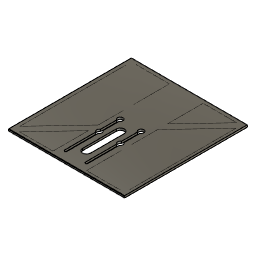
GuG_Back (Autodesk Fusion 360 design; units mm, degrees)
Autodesk Fusion 360 part; units mm, degrees
sketch "Sketch1" plane through (0, 0, 0) normal (0, 0, 1) x (1, 0, 0)
  line L0 (86.5, 91.5) -> (-86.5, 91.5)
  line L1 (-86.5, 91.5) -> (-86.5, -91.5)
  line L2 (-86.5, -91.5) -> (86.5, -91.5)
  line L3 (86.5, -91.5) -> (86.5, 91.5)
  line L4 (86.5, 91.5) -> (-86.5, -91.5) construction
  line L5 (-86.5, 91.5) -> (86.5, -91.5) construction
  line L6 (0, -91.5) -> (0, -61.5)
  line L7 (15.5, -77) -> (-15.5, -77)
  line L8 (-15.5, -77) -> (-15.5, -46)
  line L9 (-15.5, -46) -> (15.5, -46)
  line L10 (15.5, -46) -> (15.5, -77)
  line L11 (15.5, -77) -> (-15.5, -46) construction
  line L12 (-15.5, -77) -> (15.5, -46) construction
  circle A0 centre (-15.5, -77) radius 1.75
  circle A1 centre (-15.5, -46) radius 1.75
  circle A2 centre (15.5, -46) radius 1.75
  circle A3 centre (15.5, -77) radius 1.75
  line L13 (0, -61.5) -> (0, -11.5)
  line L14 (15.5, -27) -> (-15.5, -27)
  line L15 (-15.5, -27) -> (-15.5, 4)
  line L16 (-15.5, 4) -> (15.5, 4)
  line L17 (15.5, 4) -> (15.5, -27)
  line L18 (15.5, -27) -> (-15.5, 4) construction
  line L19 (-15.5, -27) -> (15.5, 4) construction
  circle A4 centre (-15.5, 4) radius 1.75
  circle A5 centre (15.5, 4) radius 1.75
  circle A6 centre (15.5, -27) radius 1.75
  circle A7 centre (-15.5, -27) radius 1.75
  circle A8 centre (-15.5, 4) radius 4
  circle A9 centre (15.5, 4) radius 4
  circle A10 centre (0, -61.5) radius 6
  circle A11 centre (0, -11.5) radius 6
  line L20 (13.75, 4) -> (17.25, 4)
  line L21 (17.25, 4) -> (17.25, -77)
  line L22 (17.25, -77) -> (13.75, -77)
  line L23 (13.75, -77) -> (13.75, 4)
  line L24 (-13.75, 4) -> (-17.25, 4)
  line L25 (-17.25, 4) -> (-17.25, -77)
  line L26 (-17.25, -77) -> (-13.75, -77)
  line L27 (-13.75, -77) -> (-13.75, 4)
  line L28 (-6, -11.5) -> (6, -11.5)
  line L29 (6, -11.5) -> (6, -61.5)
  line L30 (6, -61.5) -> (-6, -61.5)
  line L31 (-6, -61.5) -> (-6, -11.5)
  line L32 (25, -91.5) -> (-25, -91.5)
  line L33 (-25, -91.5) -> (-25, 91.5)
  line L34 (-25, 91.5) -> (25, 91.5)
  line L35 (25, 91.5) -> (25, -91.5)
  line L36 (25, -91.5) -> (-25, 91.5) construction
  line L37 (-25, -91.5) -> (25, 91.5) construction
  line L38 (-86.5, -91.5) -> (86.5, 91.5)
  line L39 (86.5, 91.5) -> (82.8666, 94.9349)
  line L40 (82.8666, 94.9349) -> (-90.1334, -88.0651)
  line L41 (-90.1334, -88.0651) -> (-86.5, -91.5)
  line L42 (-86.5, -91.5) -> (86.5, 91.5)
  line L43 (86.5, 91.5) -> (90.1334, 88.0651)
  line L44 (90.1334, 88.0651) -> (-82.8666, -94.9349)
  line L45 (-82.8666, -94.9349) -> (-86.5, -91.5)
  line L46 (86.5, -91.5) -> (-86.5, 91.5)
  line L47 (-86.5, 91.5) -> (-82.8666, 94.9349)
  line L48 (-82.8666, 94.9349) -> (90.1334, -88.0651)
  line L49 (90.1334, -88.0651) -> (86.5, -91.5)
  line L50 (86.5, -91.5) -> (-86.5, 91.5)
  line L51 (-86.5, 91.5) -> (-90.1334, 88.0651)
  line L52 (-90.1334, 88.0651) -> (82.8666, -94.9349)
  line L53 (82.8666, -94.9349) -> (86.5, -91.5)
  line L54 (81.5, -86.5) -> (-81.5, -86.5)
  line L55 (-81.5, -86.5) -> (-81.5, 86.5)
  line L56 (-81.5, 86.5) -> (81.5, 86.5)
  line L57 (81.5, 86.5) -> (81.5, -86.5)
  line L58 (81.5, -86.5) -> (-81.5, 86.5) construction
  line L59 (-81.5, -86.5) -> (81.5, 86.5) construction
  circle A12 centre (-15.5, -27) radius 4
  circle A13 centre (15.5, -27) radius 4
  point P0 (0, -91.5)
  point P1 (0, -61.5)
  point P2 (0, -11.5)
  dimension "d1" = 173
  dimension "d2" = 183
  dimension "d3" = 30
  dimension "d4" = 31
  dimension "d5" = 31
  dimension "d6" = 3.5
  dimension "d7" = 3.5
  dimension "d8" = 3.5
  dimension "d9" = 3.5
  dimension "d10" = 50
  dimension "d11" = 31
  dimension "d12" = 31
  dimension "d13" = 3.5
  dimension "d14" = 3.5
  dimension "d15" = 3.5
  dimension "d16" = 3.5
  dimension "d17" = 8
  dimension "d18" = 8
  dimension "d19" = 12
  dimension "d20" = 12
  dimension "d21" = 3.5
  dimension "d22" = 3.5
  dimension "d31" = 50
  dimension "d32" = 5
  dimension "d33" = 5
  dimension "d34" = 5
  dimension "d35" = 5
  dimension "d36" = 163
  dimension "d37" = 173
  dimension "d42" = 8
  dimension "d43" = 8
  constraint horizontal L0
  constraint perpendicular L0 L1
  constraint parallel L0 L2
  constraint parallel L1 L3
  constraint coincident L4 origin
  constraint coincident L5 origin
  constraint midpoint L2 P0
  constraint coincident P0 L6.start
  constraint perpendicular L2 L6
  constraint horizontal L7
  constraint perpendicular L7 L8
  constraint parallel L7 L9
  constraint parallel L8 L10
  constraint coincident L11 P1
  constraint coincident L12 P1
  constraint coincident P1 L6.end
  constraint coincident L7.end L8.start
  constraint coincident L8.end L9.start
  constraint coincident L9.end L10.start
  constraint coincident L7.start L10.end
  constraint parallel L6 L13
  constraint horizontal L14
  constraint perpendicular L14 L15
  constraint parallel L14 L16
  constraint parallel L15 L17
  constraint coincident L18 P2
  constraint coincident L19 P2
  constraint coincident P2 L13.end
  constraint coincident L15.end L16.start
  constraint coincident L16.end L17.start
  constraint coincident L14.start L17.end
  constraint coincident L14.end L15.start
  constraint concentric A4 A8
  constraint concentric A5 A9
  constraint horizontal L20
  constraint vertical L21
  constraint horizontal L22
  constraint vertical L23
  constraint coincident A5 L20.start
  constraint coincident L16 L20.start
  constraint horizontal L24
  constraint vertical L25
  constraint horizontal L26
  constraint vertical L27
  constraint coincident L16 L24.start
  constraint coincident A4 L24.start
  constraint horizontal L28
  constraint vertical L29
  constraint horizontal L30
  constraint vertical L31
  constraint coincident A10 L29.end
  constraint coincident A11 L28.start
  constraint horizontal L32
  constraint perpendicular L32 L33
  constraint parallel L32 L34
  constraint parallel L33 L35
  constraint coincident L36 origin
  constraint coincident L37 origin
  constraint perpendicular L38 L39
  constraint parallel L38 L40
  constraint parallel L39 L41
  constraint perpendicular L42 L43
  constraint parallel L42 L44
  constraint parallel L43 L45
  constraint perpendicular L46 L47
  constraint parallel L46 L48
  constraint parallel L47 L49
  constraint perpendicular L50 L51
  constraint parallel L50 L52
  constraint parallel L51 L53
  constraint horizontal L54
  constraint perpendicular L54 L55
  constraint parallel L54 L56
  constraint parallel L55 L57
  constraint coincident L58 origin
  constraint coincident L59 origin
  constraint concentric A7 A12
  measures "d1" distance of L1.end L2.end
  measures "d2" distance of L0.end L1.end
  measures "d3" distance of P0 P1
  measures "d4" distance of L8.end L9.end
  measures "d5" distance of L7.end L8.end
  measures "d6" diameter of A0
  measures "d7" diameter of A1
  measures "d8" diameter of A2
  measures "d9" diameter of A3
  measures "d10" distance of P1 P2
  measures "d11" distance of L15.end L16.end
  measures "d12" distance of L14.end L15.end
  measures "d13" diameter of A4
  measures "d14" diameter of A5
  measures "d15" diameter of A6
  measures "d16" diameter of A7
  measures "d17" diameter of A8
  measures "d18" diameter of A9
  measures "d19" diameter of A10
  measures "d20" diameter of A11
  measures "d21" distance of L20.start L20.end
  measures "d22" distance of L24.start L24.end
  measures "d31" distance of L33.end L34.end
  measures "d32" distance of L1.end L40.end
  measures "d33" distance of L1.end L44.end
  measures "d34" distance of L2.end L48.end
  measures "d35" distance of L2.end L52.end
  measures "d36" distance of L55.end L56.end
  measures "d37" distance of L54.end L55.end
  measures "d42" diameter of A12
  measures "d43" diameter of A13
extrude "Extrude1" add sketch "Sketch1" along normal blind 3 contours L0 L33 L34 L35 L56 | L0 L35 L40 L56 | L0 L33 L48 L56 | L0 L38 L40 L42 L56 L57 | L35 L40 L56 | L33 L35 L40 L48 L56 | L0 L46 L48 L50 L55 L56 | L33 L48 L56 | L3 L38 L42 L44 L57 | L35 L38 L40 L42 L56 L57 | L16 L35 L38 L40 L42 L48 | L1 L46 L50 L52 L55 | L33 L46 L48 L50 L55 L56 | L16 L33 L40 L46 L48 L50 | L3 L44 L48 L57 | L35 L38 L42 L44 L57 | L16 A9 L35 L38 L42 L44 | L16 L40 L48 | L1 L40 L52 L55 | L33 L46 L50 L52 L55 | L16 A8 L33 L46 L50 L52 | L3 L46 L48 L50 L57 | L35 L44 L48 L57 | A9 L21 L35 L44 L48 | L16 L38 L42 L48 | L16 L38 L42 L44 L48 | L16 L40 L46 L50 | L16 L38 L40 L42 L46 L48 L50 | L1 L38 L40 L42 L55 | L33 L40 L52 L55 | A8 L25 L33 L40 L52 | L16 L40 L46 L50 L52 | L2 L46 L50 L52 L54 L57 | L35 L46 L48 L50 L57 | L21 L35 L46 L48 L50 | L16 A9 L44 | L16 A9 L23 L44 L48 | L38 L42 L44 L46 L48 L50 | L38 L40 L42 L46 L50 L52 | L2 L38 L42 L44 L54 L55 | L33 L38 L40 L42 L55 | L25 L33 L38 L40 L42 | L16 A8 L27 L40 L52 | L16 A8 L52 | L2 L35 L52 L54 | L35 L46 L50 L52 L54 L57 | L21 L35 L46 L50 L52 A13 | L23 L44 L46 L48 L50 | A11 L38 L42 L44 L46 L50 L52 | L27 L38 L40 L42 L52 | L2 L33 L44 L54 | L33 L38 L42 L44 L54 L55 | L25 L33 L38 L42 L44 A12 | L2 L6 L32 L35 L54 | L35 L52 L54 | L6 L7 A3 L21 L35 L52 L54 A13 | A11 L23 L29 L44 L46 L50 L52 | A11 L27 L31 L38 L42 L44 L52 | L2 L6 L32 L33 L54 | L33 L44 L54 | L6 L7 A0 L25 L33 L44 L54 A12 | L21 L52 A13 | L21 L52 A13 | L25 L44 A12 | L25 L44 A12 | L14 L23 L29 L52 A13 | L14 L27 L31 L44 A12 | L6 L7 L9 A10 L27 L31 | L6 L7 L9 A10 L23 L29 | L14 L23 A13 | L9 L14 L23 L29 A13 | L14 L23 A13 | L14 L27 A12 | L9 L14 L27 L31 A12 | L14 L27 A12
chamfer "Chamfer1" distance 0.5 angle 45 2 edges at (0, -91.5, 3) (0, -91.5, 0)
chamfer "Chamfer2" distance 0.5 angle 45 2 edges at (0, 91.5, 3) (0, 91.5, 0)
extrude "Extrude2" cut 1 faces at (86.5, 30.3333, 2) along direction (-1, 0, 0) blind 0.5
extrude "Extrude3" cut 1 faces at (-86.5, -30.3333, 2) along direction (1, 0, 0) blind 0.5
extrude "Extrude5" cut sketch "Sketch1" along normal blind 2 contours L35 L40 L56 | L33 L48 L56 | L35 L44 L48 L57 | L33 L40 L52 L55 | L35 L52 L54 | L33 L44 L54
extrude "Extrude6" cut sketch "Sketch1" along normal blind 3 contours L21 L52 A13 | L21 L52 A13 | L17 L21 L52 A13 | L25 L44 A12 | L25 L44 A12 | L15 L25 L44 A12 | L17 A6 L21 L52 | A6 L21 L23 A13 | L17 L52 A13 | L15 A7 L25 L44 | A7 L25 L27 A12 | L15 L44 A12 | L14 L17 A6 | L17 A6 L23 L52 A13 | L14 L23 A13 | L14 L23 A13 | L14 L27 A12 | L15 A7 L27 L44 A12 | L14 L15 A7 | L14 L27 A12 | L14 L17 A6 | L14 L15 A7
equation "d36 = 173.000 mm - 10 mm"
equation "d37 = 183.000 mm - 10 mm"
